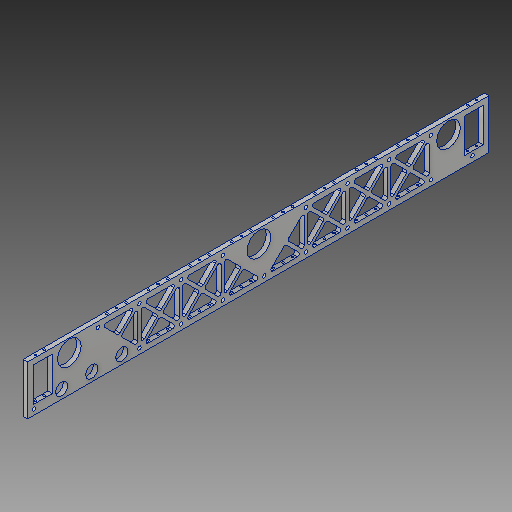
# Autodesk Inventor part: Inner Plate
Saved by Autodesk Inventor 2019.4 (Build 234330000, 330)
## iProperties
Created: 2019-12-07
Part Number: Inner Plate
Material: Aluminum 6061
Document SubType Name: Modeling
Designer: admin
Density: 2.7 g/cm^3
Appearance: Aluminum - Flat
Mass: 558.829 g
Surface Area: 1040.5 cm^2
Volume: 206.974 cm^3
Author: admin
Autodesk Inventor part; units mm, degrees
ref_plane "YZ Plane" through (0, 0, 0) normal (1, 0, 0) x (0, 1, 0)
ref_plane "XZ Plane" through (0, 0, 0) normal (0, 1, 0) x (-1, 0, 0)
sketch "Sketch1" plane through (0, 0, 0) normal (1, 0, 0) x (0, 1, 0)
  line L0 (49.2406, -203.3994) -> (-27.7594, -203.3994)
  line L1 (-27.7594, -203.3994) -> (-27.7594, -3.3994)
  line L2 (-27.7594, -3.3994) -> (49.2406, -3.3994)
  line L3 (49.2406, -3.3994) -> (49.2406, -203.3994)
  line L4 (32.2406, -193.3994) -> (32.2406, -13.3994) construction
  line L5 (32.2406, -103.3994) -> (2.7957, -103.3994) construction
  point P0 (0, 0)
  dimension "d2" = 77
  dimension "d3" = 200
  dimension "d7" = 180
  dimension "d8" = 60
  dimension "d9" = 100
  constraints: 12 end point, 2 horizontal, 2 parallel, 1 midpoint, 1 perpendicular, 1 vertical
  measures "d2" distance of L0.start L0.end
  measures "d3" distance of L2.end L0.start
  measures "d7" distance of L4.end L4.start
  measures "d8" distance between parallel lines of L1 L4
  measures "d9" distance between parallel lines of L0 L5
extrude "Extrusion1" add sketch "Sketch1" along normal blind 7
sketch "Sketch2" plane through (7, 0, 0) normal (1, 0, 0) x (0, 0, -1)
  line L0 (203.3994, 49.2406) -> (3.3994, 49.2406) projected
  line L1 (103.3994, 49.2406) -> (103.3994, -27.7594) construction
  line L2 (3.3994, -27.7594) -> (203.3994, -27.7594) projected
  circle A0 centre (103.3994, -13.7594) radius 9.5
  circle A1 centre (56.4094, -13.7594) radius 9.5
  circle A2 centre (150.3894, -13.7594) radius 9.5
  circle A3 centre (68.3994, 29.2406) radius 18.5
  point P0 (0, 0)
  dimension "d10" = 19
  dimension "d11" = 63
  dimension "d14" = 19
  dimension "d15" = 19
  dimension "d16" = 63
  dimension "d17" = 63
  dimension "d18" = 46.99
  dimension "d19" = 46.99
  dimension "d22" = 37
  dimension "d23" = 20
  dimension "d24" = 11.99
  constraints: 4 centre point, 2 end point, 2 midpoint, 1 point on line
  measures "d10" diameter of A0
  measures "d11" distance from line of L0 A0.centre
  measures "d14" diameter of A1
  measures "d15" diameter of A2
  measures "d16" distance from line of L0 A2.centre
  measures "d17" distance from line of L0 A1.centre
  measures "d18" distance of A0.centre A1.centre
  measures "d19" distance of A0.centre A2.centre
  measures "d22" diameter of A3
  measures "d23" distance from line of L0 A3.centre
  measures "d24" horizontal distance of A1.centre A3.centre
extrude "Extrusion2" cut sketch "Sketch2" against normal blind 10
sketch "Sketch3" plane through (7, 0, 0) normal (1, 0, 0) x (0, 0, -1)
  line L0 (203.3994, 49.2406) -> (3.3994, 49.2406) projected
  line L1 (203.3994, 49.2406) -> (723.3994, 49.2406)
  line L2 (723.3994, 49.2406) -> (723.3994, -27.7594)
  line L3 (723.3994, -27.7594) -> (203.3994, -27.7594)
  line L4 (203.3994, -27.7594) -> (203.3994, 49.2406)
  point P0 (0, 0)
  dimension "d25" = 520
  dimension "d26" = 77
  constraints: 8 end point, 2 parallel, 1 horizontal, 1 perpendicular
  measures "d25" distance of L2.end L3.end
  measures "d26" distance of L1.end L2.end
extrude "Extrusion3" add sketch "Sketch3" against normal blind 7
sketch "Sketch4" plane through (7, 0, 0) normal (1, 0, 0) x (0, 0, -1)
  circle A0 centre (660.3994, 28.2406) radius 18.5
  line L0 (3.3994, 49.2406) -> (723.3994, 49.2406) projected
  line L1 (723.3994, 49.2406) -> (723.3994, -27.7594) projected
  line L2 (3.3994, -27.7594) -> (723.3994, -27.7594) projected
  circle A1 centre (364.3994, 28.2406) radius 18.5
  circle A2 centre (68.3994, 29.2406) radius 18.5 projected
  point P0 (0, 0)
  dimension "d29" = 37
  dimension "d30" = 21
  dimension "d33" = 37
  dimension "d34" = 21
  dimension "d37" = 296
  dimension "d38" = 296
  constraints: 2 centre point
  measures "d29" diameter of A0
  measures "d30" distance from line of L0 A0.centre
  measures "d33" diameter of A1
  measures "d34" distance from line of L0 A1.centre
  measures "d37" horizontal distance of A2.centre A1.centre
  measures "d38" distance of A1.centre A0.centre
extrude "Extrusion4" cut sketch "Sketch4" against normal blind 7 contours A0 | A1
sketch "Sketch5" plane through (7, 0, 0) normal (1, 0, 0) x (0, 0, -1)
  line L0 (3.3994, -27.7594) -> (723.3994, -27.7594) projected
  circle A0 centre (660.3994, 28.2406) radius 18.5 projected
  line L1 (630.3994, 40.7406) -> (570.3994, 40.7406) construction
  line L2 (570.3994, 40.7406) -> (570.3994, -19.2594) construction
  line L3 (570.3994, -19.2594) -> (630.3994, -19.2594) construction
  line L4 (630.3994, -19.2594) -> (630.3994, 40.7406) construction
  line L5 (630.3994, 40.7406) -> (570.3994, -19.2594) construction
  line L6 (570.3994, 40.7406) -> (630.3994, -19.2594) construction
  line L7 (3.3994, 49.2406) -> (723.3994, 49.2406) projected
  line L8 (630.3994, -15.7239) -> (630.3994, 37.205)
  line L9 (626.8639, 40.7406) -> (573.9349, 40.7406)
  line L10 (570.3994, 37.205) -> (570.3994, -15.7239)
  line L11 (573.9349, -19.2594) -> (626.8639, -19.2594)
  line L12 (630.3994, -15.7239) -> (603.9349, 10.7406)
  line L13 (600.3994, 14.2761) -> (573.9349, 40.7406)
  line L14 (626.8639, -19.2594) -> (600.3994, 7.205)
  line L15 (596.8639, 10.7406) -> (570.3994, 37.205)
  line L16 (573.9349, -19.2594) -> (600.3994, 7.205)
  line L17 (603.9349, 10.7406) -> (630.3994, 37.205)
  line L18 (570.3994, -15.7239) -> (596.8639, 10.7406)
  line L19 (600.3994, 14.2761) -> (626.8639, 40.7406)
  line L20 (505.3994, -15.7239) -> (531.8639, 10.7406)
  line L21 (508.9349, -19.2594) -> (535.3994, 7.205)
  line L22 (561.8639, -19.2594) -> (535.3994, 7.205)
  line L23 (508.9349, -19.2594) -> (561.8639, -19.2594)
  line L24 (505.3994, 37.205) -> (505.3994, -15.7239)
  line L25 (531.8639, 10.7406) -> (505.3994, 37.205)
  line L26 (535.3994, 14.2761) -> (508.9349, 40.7406)
  line L27 (561.8639, 40.7406) -> (508.9349, 40.7406)
  line L28 (535.3994, 14.2761) -> (561.8639, 40.7406)
  line L29 (538.9349, 10.7406) -> (565.3994, 37.205)
  line L30 (565.3994, -19.2594) -> (565.3994, 40.7406) construction
  line L31 (565.3994, -15.7239) -> (565.3994, 37.205)
  line L32 (565.3994, -15.7239) -> (538.9349, 10.7406)
  line L33 (440.3994, -15.7239) -> (466.8639, 10.7406)
  line L34 (443.9349, -19.2594) -> (470.3994, 7.205)
  line L35 (496.8639, -19.2594) -> (470.3994, 7.205)
  line L36 (443.9349, -19.2594) -> (496.8639, -19.2594)
  line L37 (440.3994, 37.205) -> (440.3994, -15.7239)
  line L38 (466.8639, 10.7406) -> (440.3994, 37.205)
  line L39 (470.3994, 14.2761) -> (443.9349, 40.7406)
  line L40 (496.8639, 40.7406) -> (443.9349, 40.7406)
  line L41 (470.3994, 14.2761) -> (496.8639, 40.7406)
  line L42 (473.9349, 10.7406) -> (500.3994, 37.205)
  line L43 (500.3994, -19.2594) -> (500.3994, 40.7406) construction
  line L44 (500.3994, -15.7239) -> (500.3994, 37.205)
  line L45 (500.3994, -15.7239) -> (473.9349, 10.7406)
  line L46 (375.3994, -15.7239) -> (401.8639, 10.7406)
  line L47 (378.9349, -19.2594) -> (405.3994, 7.205)
  line L48 (431.8639, -19.2594) -> (405.3994, 7.205)
  line L49 (378.9349, -19.2594) -> (431.8639, -19.2594)
  line L50 (375.3994, 37.205) -> (375.3994, -15.7239)
  line L51 (401.8639, 10.7406) -> (375.3994, 37.205)
  line L52 (405.3994, 14.2761) -> (378.9349, 40.7406)
  line L53 (431.8639, 40.7406) -> (378.9349, 40.7406)
  line L54 (405.3994, 14.2761) -> (431.8639, 40.7406)
  line L55 (408.9349, 10.7406) -> (435.3994, 37.205)
  line L56 (435.3994, -19.2594) -> (435.3994, 40.7406) construction
  line L57 (435.3994, -15.7239) -> (435.3994, 37.205)
  line L58 (435.3994, -15.7239) -> (408.9349, 10.7406)
  line L59 (310.3994, -15.7239) -> (336.8639, 10.7406)
  line L60 (313.9349, -19.2594) -> (340.3994, 7.205)
  line L61 (366.8639, -19.2594) -> (340.3994, 7.205)
  line L62 (313.9349, -19.2594) -> (366.8639, -19.2594)
  line L63 (310.3994, 37.205) -> (310.3994, -15.7239)
  line L64 (336.8639, 10.7406) -> (310.3994, 37.205)
  line L65 (340.3994, 14.2761) -> (313.9349, 40.7406)
  line L66 (366.8639, 40.7406) -> (313.9349, 40.7406)
  line L67 (340.3994, 14.2761) -> (366.8639, 40.7406)
  line L68 (343.9349, 10.7406) -> (370.3994, 37.205)
  line L69 (370.3994, -19.2594) -> (370.3994, 40.7406) construction
  line L70 (370.3994, -15.7239) -> (370.3994, 37.205)
  line L71 (370.3994, -15.7239) -> (343.9349, 10.7406)
  line L72 (245.3994, -15.7239) -> (271.8639, 10.7406)
  line L73 (248.9349, -19.2594) -> (275.3994, 7.205)
  line L74 (301.8639, -19.2594) -> (275.3994, 7.205)
  line L75 (248.9349, -19.2594) -> (301.8639, -19.2594)
  line L76 (245.3994, 37.205) -> (245.3994, -15.7239)
  line L77 (271.8639, 10.7406) -> (245.3994, 37.205)
  line L78 (275.3994, 14.2761) -> (248.9349, 40.7406)
  line L79 (301.8639, 40.7406) -> (248.9349, 40.7406)
  line L80 (275.3994, 14.2761) -> (301.8639, 40.7406)
  line L81 (278.9349, 10.7406) -> (305.3994, 37.205)
  line L82 (305.3994, -19.2594) -> (305.3994, 40.7406) construction
  line L83 (305.3994, -15.7239) -> (305.3994, 37.205)
  line L84 (305.3994, -15.7239) -> (278.9349, 10.7406)
  line L85 (180.3994, -15.7239) -> (206.8639, 10.7406)
  line L86 (183.9349, -19.2594) -> (210.3994, 7.205)
  line L87 (236.8639, -19.2594) -> (210.3994, 7.205)
  line L88 (183.9349, -19.2594) -> (236.8639, -19.2594)
  line L89 (180.3994, 37.205) -> (180.3994, -15.7239)
  line L90 (206.8639, 10.7406) -> (180.3994, 37.205)
  line L91 (210.3994, 14.2761) -> (183.9349, 40.7406)
  line L92 (236.8639, 40.7406) -> (183.9349, 40.7406)
  line L93 (210.3994, 14.2761) -> (236.8639, 40.7406)
  line L94 (213.9349, 10.7406) -> (240.3994, 37.205)
  line L95 (240.3994, -19.2594) -> (240.3994, 40.7406) construction
  line L96 (240.3994, -15.7239) -> (240.3994, 37.205)
  line L97 (240.3994, -15.7239) -> (213.9349, 10.7406)
  line L98 (115.3994, -15.7239) -> (141.8639, 10.7406)
  line L99 (118.9349, -19.2594) -> (145.3994, 7.205)
  line L100 (171.8639, -19.2594) -> (145.3994, 7.205)
  line L101 (118.9349, -19.2594) -> (171.8639, -19.2594)
  line L102 (115.3994, 37.205) -> (115.3994, -15.7239)
  line L103 (141.8639, 10.7406) -> (115.3994, 37.205)
  line L104 (145.3994, 14.2761) -> (118.9349, 40.7406)
  line L105 (171.8639, 40.7406) -> (118.9349, 40.7406)
  line L106 (145.3994, 14.2761) -> (171.8639, 40.7406)
  line L107 (148.9349, 10.7406) -> (175.3994, 37.205)
  line L108 (175.3994, -19.2594) -> (175.3994, 40.7406) construction
  line L109 (175.3994, -15.7239) -> (175.3994, 37.205)
  line L110 (175.3994, -15.7239) -> (148.9349, 10.7406)
  circle A1 centre (567.8994, -19.2594) radius 2.75
  circle A2 centre (567.8994, 40.7406) radius 2.75
  circle A3 centre (502.8994, -19.2594) radius 2.75
  circle A4 centre (502.8994, 40.7406) radius 2.75
  circle A5 centre (437.8994, -19.2594) radius 2.75
  circle A6 centre (437.8994, 40.7406) radius 2.75
  circle A7 centre (372.8994, -19.2594) radius 2.75
  circle A8 centre (372.8994, 40.7406) radius 2.75
  circle A9 centre (307.8994, -19.2594) radius 2.75
  circle A10 centre (307.8994, 40.7406) radius 2.75
  circle A11 centre (242.8994, -19.2594) radius 2.75
  circle A12 centre (242.8994, 40.7406) radius 2.75
  circle A13 centre (177.8994, -19.2594) radius 2.75
  circle A14 centre (177.8994, 40.7406) radius 2.75
  circle A15 centre (112.8994, -19.2594) radius 2.75
  circle A16 centre (112.8994, 40.7406) radius 2.75
  circle A17 centre (632.8994, -19.2594) radius 2.75
  circle A18 centre (632.8994, 40.7406) radius 2.75
  circle A19 centre (567.8994, -19.2594) radius 2.75
  circle A20 centre (567.8994, 40.7406) radius 2.75
  circle A21 centre (502.8994, -19.2594) radius 2.75
  circle A22 centre (502.8994, 40.7406) radius 2.75
  circle A23 centre (437.8994, -19.2594) radius 2.75
  circle A24 centre (437.8994, 40.7406) radius 2.75
  circle A25 centre (372.8994, -19.2594) radius 2.75
  circle A26 centre (372.8994, 40.7406) radius 2.75
  circle A27 centre (307.8994, -19.2594) radius 2.75
  circle A28 centre (307.8994, 40.7406) radius 2.75
  circle A29 centre (242.8994, -19.2594) radius 2.75
  circle A30 centre (242.8994, 40.7406) radius 2.75
  circle A31 centre (177.8994, -19.2594) radius 2.75
  circle A32 centre (177.8994, 40.7406) radius 2.75
  point P0 (0, 0)
  point P1 (600.3994, 10.7406)
  point P2 (68.3994, 49.2406)
  point P3 (658.3994, 49.2406)
  dimension "d44" = 60
  dimension "d45" = 60
  dimension "d50" = 30
  dimension "d51" = 8.5
  dimension "d52" = 2.5
  dimension "d53" = 2.5
  dimension "d54" = 2.5
  dimension "d55" = 2.5
  dimension "d56" = 2.5
  dimension "d57" = 2.5
  dimension "d58" = 2.5
  dimension "d59" = 2.5
  dimension "d64" = 65
  dimension "d70" = 5.5
  dimension "d71" = 5.5
  dimension "d72" = 2.5
  dimension "d73" = 2.5
  dimension "d74" = 8.5
  dimension "d75" = 8.5
  dimension "d78" = 65
  dimension "d81" = 65
  constraints: 218 end point, 32 centre point, 22 point on line, 10 parallel, 4 horizontal, 3 collinear, 2 midpoint, 1 perpendicular, 248 other
  measures "d44" distance of L3.end L2.end
  measures "d45" distance of L2.end L1.end
  measures "d50" distance from line of A0.centre L4
  measures "d51" distance between parallel lines of L7 L1
  measures "d52" distance between parallel lines of L5 L17
  measures "d53" distance between parallel lines of L5 L19
  measures "d54" distance between parallel lines of L6 L12
  measures "d55" distance between parallel lines of L6 L14
  measures "d56" distance between parallel lines of L5 L18
  measures "d57" distance between parallel lines of L5 L16
  measures "d58" distance between parallel lines of L6 L13
  measures "d59" distance between parallel lines of L6 L15
  measures "d64" distance of L10.end L20.start
  measures "d70" diameter of A1
  measures "d71" diameter of A2
  measures "d72" distance from line of L10 A2.centre
  measures "d73" distance from line of L10 A1.centre
  measures "d74" distance from line of L0 A1.centre
  measures "d75" distance from line of L7 A2.centre
  measures "d78" distance of A1.centre A3.centre
  measures "d81" distance of A1.centre A17.centre
extrude "Extrusion5" cut sketch "Sketch5" against normal blind 10 contours L12 L17 L8 | L19 L13 L9 | L15 L18 L10 | L16 L14 L11 | L24 L25 L20 | L21 L22 L23 | L26 L27 L28 | L29 L31 L32 | L37 L38 L33 | L34 L35 L36 | L39 L40 L41 | L42 L44 L45 | L47 L48 L49 | L55 L57 L58 | L63 L64 L59 | L60 L61 L62 | L76 L77 L72 | L73 L74 L75 | L78 L79 L80 | L81 L83 L84 | L89 L90 L85 | L86 L87 L88 | L91 L92 L93 | L94 L96 L97 | L104 L105 L106 | L107 L109 L110 | A1 | A2 | A3 | A4 | A5 | A6 | A7 | A9 | A10 | A11 | A12 | A13 | A14 | A16 | A17 | A18
fillet "Fillet2" radius 3 78 edges at (3.5, 40.7406, -626.8639) (3.5, 37.205, -630.3994) (3.5, 7.205, -600.3994) (3.5, 10.7406, -603.9349) (3.5, 10.7406, -596.8639) (3.5, 14.2761, -600.3994) (3.5, -19.2594, -626.8639) (3.5, -15.7239, -630.3994) (3.5, -15.7239, -565.3994) (3.5, -19.2594, -561.8639) (3.5, -19.2594, -573.9349) (3.5, -15.7239, -570.3994) (3.5, 37.205, -565.3994) (3.5, 40.7406, -561.8639) (3.5, 37.205, -570.3994) (3.5, 40.7406, -573.9349) (3.5, 10.7406, -538.9349) (3.5, 7.205, -535.3994) (3.5, 10.7406, -531.8639) (3.5, 14.2761, -535.3994) (3.5, -15.7239, -500.3994) (3.5, -19.2594, -496.8639) (3.5, -15.7239, -505.3994) (3.5, -19.2594, -508.9349) (3.5, 37.205, -500.3994) (3.5, 40.7406, -496.8639) (3.5, 37.205, -505.3994) (3.5, 40.7406, -508.9349) (3.5, 10.7406, -473.9349) (3.5, 7.205, -470.3994) (3.5, 10.7406, -466.8639) (3.5, 14.2761, -470.3994) (3.5, 37.205, -440.3994) (3.5, 40.7406, -443.9349) (3.5, 37.205, -435.3994) (3.5, -19.2594, -443.9349) (3.5, -15.7239, -440.3994) (3.5, -15.7239, -435.3994) (3.5, -19.2594, -431.8639) (3.5, 10.7406, -408.9349) (3.5, 7.205, -405.3994) (3.5, -19.2594, -366.8639) (3.5, -19.2594, -378.9349) (3.5, 10.7406, -336.8639) (3.5, 7.205, -340.3994) (3.5, 37.205, -310.3994) (3.5, 37.205, -305.3994) (3.5, 40.7406, -301.8639) (3.5, -19.2594, -301.8639) (3.5, -15.7239, -310.3994) (3.5, -15.7239, -305.3994) (3.5, -19.2594, -313.9349) (3.5, 10.7406, -278.9349) (3.5, 7.205, -275.3994) (3.5, 14.2761, -275.3994) (3.5, 10.7406, -271.8639) (3.5, -15.7239, -240.3994) (3.5, -19.2594, -248.9349) (3.5, -15.7239, -245.3994) (3.5, -19.2594, -236.8639) (3.5, 37.205, -245.3994) (3.5, 40.7406, -236.8639) (3.5, 40.7406, -248.9349) (3.5, 37.205, -240.3994) (3.5, 10.7406, -213.9349) (3.5, 7.205, -210.3994) (3.5, 10.7406, -206.8639) (3.5, 14.2761, -210.3994) (3.5, -19.2594, -183.9349) (3.5, -15.7239, -180.3994) (3.5, -15.7239, -175.3994) (3.5, 37.205, -180.3994) (3.5, 40.7406, -171.8639) (3.5, 37.205, -175.3994) (3.5, 40.7406, -183.9349) (3.5, 14.2761, -145.3994) (3.5, 10.7406, -148.9349) (3.5, 40.7406, -118.9349)
sketch "Sketch6" plane through (0, 0, 0) normal (-1, 0, 0) x (0, 0, 1)
  circle A0 centre (-697.8994, -19.2594) radius 2.75
  line L0 (-723.3994, -27.7594) -> (-3.3994, -27.7594) projected
  circle A1 centre (-632.8994, -19.2594) radius 2.75 projected
  circle A2 centre (-13.3994, -19.2594) radius 2.75
  line L1 (-3.3994, 49.2406) -> (-3.3994, -27.7594) projected
  point P0 (0, 0)
  point P1 (-702.6826, -27.7594)
  point P2 (-3.3994, -15.7594)
  dimension "d85" = 5.5
  dimension "d86" = 8.5
  dimension "d87" = 65
  dimension "d90" = 5.5
  dimension "d91" = 10
  dimension "d92" = 8.5
  constraints: 2 centre point
  measures "d85" diameter of A0
  measures "d86" distance from line of L0 A0.centre
  measures "d87" distance of A1.centre A0.centre
  measures "d90" diameter of A2
  measures "d91" distance from line of L1 A2.centre
  measures "d92" distance from line of L0 A2.centre
extrude "Extrusion6" cut sketch "Sketch6" against normal blind 10 contours A0 | A2
sketch "Sketch7" plane through (0, -27.7594, -723.3994) normal (0, -1, 0) x (1, 0, 0)
  line L0 (7, 532.2218) -> (0, 532.2218) projected
  line L1 (7, 493.7782) -> (7, 532.2218) projected
  line L2 (0, 493.7782) -> (7, 493.7782) projected
  line L3 (0, 532.2218) -> (0, 493.7782) projected
  circle A0 centre (3.5, 513) radius 1.65
  circle A1 centre (3.5, 498) radius 1.65
  circle A2 centre (3.5, 528) radius 1.65
  line L4 (3.5, 513) -> (7, 513) construction
  circle A3 centre (3.5, 463) radius 1.65
  circle A4 centre (3.5, 448) radius 1.65
  circle A5 centre (3.5, 433) radius 1.65
  circle A6 centre (3.5, 398) radius 1.65
  circle A7 centre (3.5, 383) radius 1.65
  circle A8 centre (3.5, 368) radius 1.65
  circle A9 centre (3.5, 333) radius 1.65
  circle A10 centre (3.5, 318) radius 1.65
  circle A11 centre (3.5, 303) radius 1.65
  circle A12 centre (3.5, 268) radius 1.65
  circle A13 centre (3.5, 253) radius 1.65
  circle A14 centre (3.5, 238) radius 1.65
  circle A15 centre (3.5, 203) radius 1.65
  circle A16 centre (3.5, 188) radius 1.65
  circle A17 centre (3.5, 173) radius 1.65
  circle A18 centre (3.5, 138) radius 1.65
  circle A19 centre (3.5, 123) radius 1.65
  circle A20 centre (3.5, 108) radius 1.65
  point P0 (0, 723.3994)
  dimension "d93" = 3.3
  dimension "d94" = 3.3
  dimension "d95" = 3.3
  dimension "d96" = 15
  dimension "d97" = 15
  dimension "d98" = 15
  dimension "d99" = 15
  dimension "d100" = 3.5
  dimension "d103" = 65
  constraints: 21 centre point, 2 end point, 1 midpoint, 1 perpendicular, 1 vertical, 36 other
  measures "d93" diameter of A0
  measures "d94" diameter of A1
  measures "d95" diameter of A2
  measures "d96" distance of L4.start A2.centre
  measures "d97" distance of A1.centre L4.start
  measures "d98" distance of A1.centre L4.start
  measures "d99" distance of L4.start A2.centre
  measures "d100" distance from line of L3 L4.start
  measures "d103" distance of A2.centre A3.centre
extrude "Extrusion7" cut sketch "Sketch7" against normal up to surface (8.5 mm away) contours A0 | A1 | A2 | A3 | A4 | A5 | A6 | A7 | A8 | A9 | A10 | A11 | A12 | A13 | A14 | A15 | A16 | A17 | A18 | A19 | A20
sketch "Sketch8" plane through (0, 49.2406, -3.3994) normal (0, 1, 0) x (1, 0, 0)
  circle A0 centre (3.5, 192) radius 1.65 projected
  circle A1 centre (3.5, 207) radius 1.65 projected
  circle A2 centre (3.5, 222) radius 1.65 projected
  circle A3 centre (3.5, 192) radius 1.65
  circle A4 centre (3.5, 207) radius 1.65
  circle A5 centre (3.5, 222) radius 1.65
  line L0 (0, 0) -> (0, 720) projected
  circle A6 centre (3.5, 127) radius 1.65
  circle A7 centre (3.5, 142) radius 1.65
  circle A8 centre (3.5, 157) radius 1.65
  circle A9 centre (3.5, 257) radius 1.65
  circle A10 centre (3.5, 272) radius 1.65
  circle A11 centre (3.5, 287) radius 1.65
  circle A12 centre (3.5, 322) radius 1.65
  circle A13 centre (3.5, 337) radius 1.65
  circle A14 centre (3.5, 352) radius 1.65
  circle A15 centre (3.5, 387) radius 1.65
  circle A16 centre (3.5, 402) radius 1.65
  circle A17 centre (3.5, 417) radius 1.65
  circle A18 centre (3.5, 452) radius 1.65
  circle A19 centre (3.5, 467) radius 1.65
  circle A20 centre (3.5, 482) radius 1.65
  circle A21 centre (3.5, 517) radius 1.65
  circle A22 centre (3.5, 532) radius 1.65
  circle A23 centre (3.5, 547) radius 1.65
  circle A24 centre (3.5, 582) radius 1.65
  circle A25 centre (3.5, 597) radius 1.65
  circle A26 centre (3.5, 612) radius 1.65
  point P0 (0, -3.3994)
  dimension "d112" = 65
  dimension "d119" = 65
  constraints: 24 centre point, 3 coincident, 3 concentric, 2 vertical, 42 other
  measures "d112" distance of A3.centre A6.centre
  measures "d119" distance of A3.centre A9.centre
extrude "Extrusion8" cut sketch "Sketch8" against normal up to surface (8.5 mm away)
sketch "Sketch9" plane through (0, 0, 0) normal (-1, 0, 0) x (0, 0, 1)
  line L0 (-11.8994, -12.7594) -> (-41.8994, -12.7594)
  line L1 (-41.8994, -12.7594) -> (-41.8994, 40.7406)
  line L2 (-41.8994, 40.7406) -> (-11.8994, 40.7406)
  line L3 (-11.8994, 40.7406) -> (-11.8994, -12.7594)
  line L4 (-684.8994, -12.7594) -> (-714.8994, -12.7594)
  line L5 (-714.8994, -12.7594) -> (-714.8994, 40.7406)
  line L6 (-714.8994, 40.7406) -> (-684.8994, 40.7406)
  line L7 (-684.8994, 40.7406) -> (-684.8994, -12.7594)
  line L8 (-3.3994, -27.7594) -> (-3.3994, 49.2406) projected
  line L9 (-3.3994, 49.2406) -> (-723.3994, 49.2406) projected
  line L10 (-723.3994, -27.7594) -> (-3.3994, -27.7594) projected
  line L11 (-723.3994, 49.2406) -> (-723.3994, -27.7594) projected
  point P0 (0, 0)
  dimension "d126" = 8.5
  dimension "d127" = 8.5
  dimension "d128" = 15
  dimension "d129" = 30
  dimension "d130" = 30
  dimension "d131" = 8.5
  dimension "d132" = 8.5
  dimension "d133" = 15
  constraints: 16 end point, 4 parallel, 2 horizontal, 2 perpendicular
  measures "d126" distance between parallel lines of L8 L3
  measures "d127" distance between parallel lines of L9 L2
  measures "d128" distance between parallel lines of L10 L0
  measures "d129" distance between parallel lines of L3 L1
  measures "d130" distance of L5.end L6.end
  measures "d131" distance between parallel lines of L11 L5
  measures "d132" distance between parallel lines of L9 L6
  measures "d133" distance between parallel lines of L10 L4
extrude "Extrusion9" cut sketch "Sketch9" against normal through all contours L0 L1 L2 L3 | L4 L5 L6 L7
sketch "Sketch10" plane through (0, 40.7406, -41.8994) normal (0, -1, 0) x (1, 0, 0)
  line L0 (7, 30) -> (7, 0) projected
  line L1 (0, 30) -> (7, 30) projected
  line L2 (0, 0) -> (0, 30) projected
  line L3 (0, 0) -> (7, 0) projected
  circle A0 centre (3.5, 23) radius 1.65
  circle A1 centre (3.5, 9) radius 1.65
  point P0 (0, 41.8994)
  dimension "d136" = 3.3
  dimension "d137" = 3.3
  dimension "d138" = 7
  dimension "d139" = 14
  dimension "d140" = 3.5
  dimension "d141" = 3.5
  constraints: 2 centre point
  measures "d136" diameter of A0
  measures "d137" diameter of A1
  measures "d138" distance from line of L1 A0.centre
  measures "d139" distance of A1.centre A0.centre
  measures "d140" distance from line of L0 A1.centre
  measures "d141" distance from line of L0 A0.centre
extrude "Extrusion10" cut sketch "Sketch10" along normal through all both and the other way through all contours A0 | A1
ref_plane "Work Plane1" through (0, -12.7594, -363.3994) normal (0, 0, -1) x (-1, 0, 0)
mirror "Mirror1" about plane through (0, -12.7594, -363.3994) normal (0, 0, -1) of "Extrusion10"
equation "\"d9\" = 0.5 * d3"
equation "\"d11\" = d17"
equation "\"d16\" = d17"
body "Solid1"
